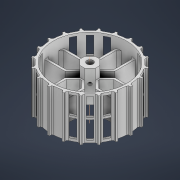
# Autodesk Inventor part: Reifen_v2
Saved by Autodesk Inventor 2021 (Build 250183000, 183)
## iProperties
Created: 2021-01-03
Part Number: Reifen_v2
Material: Generisch
Document SubType Name: Modeling
Designer: Ctroi
Density: 1 g/cm^3
Appearance: Vorgabe
Author: Ctroi
## iProperties of the stored document _3D-Druck.ipt
Created: 2021-01-03
Part Number: _3D-Druck
Material: Generisch
Document SubType Name: Modeling
Designer: Ctroi
Density: 1 g/cm^3
Appearance: Vorgabe
Author: Ctroi
Autodesk Inventor part; units mm, degrees
ref_plane "YZ Plane" through (0, 0, 0) normal (1, 0, 0) x (0, 1, 0)
ref_plane "XZ Plane" through (0, 0, 0) normal (0, 1, 0) x (-1, 0, 0)
ref_plane "XY Plane" through (0, 0, 0) normal (0, 0, 1) x (1, 0, 0)
sketch "Grundskizze" plane through (0, 0, 0) normal (0, 1, 0) x (-1, 0, 0)
  circle A0 centre (0, 0) radius 55
  circle A1 centre (0, 0) radius 52
  circle A2 centre (0, 0) radius 4.5
  line L0 (11, -3.1421) -> (3.1421, -11)
  line L1 (-3.1421, -11) -> (-11, -3.1421)
  line L2 (-11, 3.1421) -> (-3.1421, 11)
  line L3 (3.1421, 11) -> (11, 3.1421)
  line L4 (0, -77) -> (0, 77) projected
  line L5 (77, 0) -> (-77, 0) projected
  line L6 (3.1421, -11) -> (-3.1421, -11)
  line L7 (-11, -3.1421) -> (-11, 3.1421)
  line L8 (-3.1421, 11) -> (3.1421, 11)
  line L9 (11, 3.1421) -> (11, -3.1421)
  line L10 (3.1421, -11) -> (13.7487, -21.6066)
  line L11 (3.1421, -11) -> (18.1421, -11) construction
  line L12 (13.7487, -21.6066) -> (13.7487, -50.1495)
  line L13 (-3.1421, -11) -> (-13.7487, -21.6066)
  line L14 (-3.1421, -11) -> (11.8579, -11) construction
  line L15 (-13.7487, -21.6066) -> (-13.7487, -50.1495)
  line L16 (10.7487, -44.9441) -> (10.7487, -22.8492)
  line L17 (10.7487, -22.8492) -> (1.0208, -13.1213)
  line L18 (-10.7487, -44.4688) -> (-10.7487, -22.8492)
  line L19 (-10.7487, -22.8492) -> (-1.0208, -13.1213)
  line L20 (1.0208, -13.1213) -> (-1.0208, -13.1213)
  line L21 (10.7487, -44.9441) -> (10.7487, -50.877)
  line L22 (-10.7487, -44.4688) -> (-10.7487, -50.877)
  line L23 (21.6066, -13.7487) -> (50.1495, -13.7487)
  line L24 (44.4688, -10.7487) -> (50.877, -10.7487)
  line L25 (44.4688, -10.7487) -> (22.8492, -10.7487)
  line L26 (22.8492, -10.7487) -> (13.1213, -1.0208)
  line L27 (11, -3.1421) -> (21.6066, -13.7487)
  line L28 (22.8492, 10.7487) -> (13.1213, 1.0208)
  line L29 (13.1213, 1.0208) -> (13.1213, -1.0208)
  line L30 (11, 3.1421) -> (21.6066, 13.7487)
  line L31 (44.9441, 10.7487) -> (22.8492, 10.7487)
  line L32 (21.6066, 13.7487) -> (50.1495, 13.7487)
  line L33 (44.9441, 10.7487) -> (50.877, 10.7487)
  line L34 (13.7487, 21.6066) -> (13.7487, 50.1495)
  line L35 (10.7487, 44.4688) -> (10.7487, 50.877)
  line L36 (10.7487, 44.4688) -> (10.7487, 22.8492)
  line L37 (10.7487, 22.8492) -> (1.0208, 13.1213)
  line L38 (3.1421, 11) -> (13.7487, 21.6066)
  line L39 (-10.7487, 22.8492) -> (-1.0208, 13.1213)
  line L40 (-1.0208, 13.1213) -> (1.0208, 13.1213)
  line L41 (-3.1421, 11) -> (-13.7487, 21.6066)
  line L42 (-10.7487, 44.9441) -> (-10.7487, 22.8492)
  line L43 (-13.7487, 21.6066) -> (-13.7487, 50.1495)
  line L44 (-10.7487, 44.9441) -> (-10.7487, 50.877)
  line L45 (-21.6066, 13.7487) -> (-50.1495, 13.7487)
  line L46 (-44.4688, 10.7487) -> (-50.877, 10.7487)
  line L47 (-44.4688, 10.7487) -> (-22.8492, 10.7487)
  line L48 (-22.8492, 10.7487) -> (-13.1213, 1.0208)
  line L49 (-11, 3.1421) -> (-21.6066, 13.7487)
  line L50 (-22.8492, -10.7487) -> (-13.1213, -1.0208)
  line L51 (-13.1213, -1.0208) -> (-13.1213, 1.0208)
  line L52 (-11, -3.1421) -> (-21.6066, -13.7487)
  line L53 (-44.9441, -10.7487) -> (-22.8492, -10.7487)
  line L54 (-21.6066, -13.7487) -> (-50.1495, -13.7487)
  line L55 (-44.9441, -10.7487) -> (-50.877, -10.7487)
  line L56 (-10.7487, -47.6729) -> (-7.4827, -51.4588)
  line L57 (-7.4827, -51.4588) -> (-10.7487, -51.4588)
  line L58 (-10.7487, -51.4588) -> (-10.7487, -47.6729)
  line L59 (10.7487, -47.6729) -> (7.4827, -51.4588)
  line L60 (7.4827, -51.4588) -> (10.7487, -51.4588)
  line L61 (10.7487, -51.4588) -> (10.7487, -47.6729)
  line L62 (51.4588, -10.7487) -> (47.6729, -10.7487)
  line L63 (47.6729, -10.7487) -> (51.4588, -7.4827)
  line L64 (51.4588, -7.4827) -> (51.4588, -10.7487)
  line L65 (51.4588, 10.7487) -> (47.6729, 10.7487)
  line L66 (47.6729, 10.7487) -> (51.4588, 7.4827)
  line L67 (51.4588, 7.4827) -> (51.4588, 10.7487)
  circle A3 centre (0, 0) radius 4.5
  line L68 (10.7487, 51.4588) -> (10.7487, 47.6729)
  line L69 (10.7487, 47.6729) -> (7.4827, 51.4588)
  line L70 (7.4827, 51.4588) -> (10.7487, 51.4588)
  line L71 (-10.7487, 51.4588) -> (-10.7487, 47.6729)
  line L72 (-10.7487, 47.6729) -> (-7.4827, 51.4588)
  line L73 (-7.4827, 51.4588) -> (-10.7487, 51.4588)
  circle A4 centre (0, 0) radius 4.5
  line L74 (-51.4588, 10.7487) -> (-47.6729, 10.7487)
  line L75 (-47.6729, 10.7487) -> (-51.4588, 7.4827)
  line L76 (-51.4588, 7.4827) -> (-51.4588, 10.7487)
  line L77 (-51.4588, -10.7487) -> (-47.6729, -10.7487)
  line L78 (-47.6729, -10.7487) -> (-51.4588, -7.4827)
  line L79 (-51.4588, -7.4827) -> (-51.4588, -10.7487)
  circle A5 centre (0, 0) radius 4.5
  point P0 (0, -11)
  point P1 (-50.1495, 13.7487)
  point P2 (-50.877, 10.7487)
  point P3 (-50.1495, -13.7487)
  point P4 (13.7487, 50.1495)
  point P5 (10.7487, 50.877)
  point P6 (-13.7487, 50.1495)
  point P7 (50.877, -10.7487)
  point P8 (50.877, 10.7487)
  point P9 (50.1495, 13.7487)
  point P10 (50.877, 10.7487)
  point P11 (10.7487, 50.877)
  point P12 (-10.7487, 50.877)
  point P13 (-50.877, 10.7487)
  point P14 (-50.877, -10.7487)
  dimension "d0" = 110
  dimension "d1" = 3
  dimension "d2" = 9
  dimension "d7" = 15
  dimension "d8" = 45
  dimension "d10" = 135
  dimension "d11" = 3
  dimension "d12" = 3
  dimension "d52" = 360
  dimension "d88" = 5
  dimension "d91" = 360
  dimension "d93" = 40.784
  constraints: 156 end point, 6 centre point, 6 vertical, 5 horizontal, 5 point on circle, 4 coincident, 4 parallel, 4 perpendicular, 3 symmetric about line, 2 equal length, 2 midpoint, 1 point on line, 174 other
  measures "d0" diameter of A0
  measures "d1" radial gap between concentric circles of A0 A1
  measures "d2" diameter of A2
  measures "d7" distance of L0.end L10.end
  measures "d8" angle of L10 L11
  measures "d10" angle of L13 L14
  measures "d11" distance between parallel lines of L12 L16
  measures "d12" distance between parallel lines of L15 L18
  measures "d88" distance of L56.start L56.end
  measures "d93" angle of L56 L22
extrude "Außenrahmen" add sketch "Grundskizze" along normal blind 45 and the other way blind 15 contours L5 A1 L67 L65 L68 L70 L4 A0 | A0 L4 A1 L60 L61 L62 L64 L5 | L4 A1 L73 L71 L74 L76 L5 A0 | A0 L5 A1 L79 L77 L58 L57 L4 | A1 L65 L67 | L64 L62 A1 | L70 L68 A1 | A1 L71 L73 | L57 L58 A1 | A1 L61 L60 | L76 L74 A1 | A1 L77 L79
extrude "Radnabe" add sketch "Grundskizze" along normal blind 45 contours L9 L0 L6 L4 A2 L5 | L5 A2 L4 L8 L3 L9 | L4 A2 L5 L7 L2 L8 | L6 L1 L7 L5 A2 L4
sketch "Profilskizze" plane through (0, 45, 0) normal (0, 1, 0) x (1, 0, 0)
  circle A0 centre (0, 0) radius 55 projected
  circle A1 centre (0, 0) radius 55 projected
  line L0 (1.5, 54.9795) -> (1.5, 58.5)
  line L1 (1, 59) -> (-1, 59)
  line L2 (-1.5, 58.5) -> (-1.5, 54.9795)
  line L3 (0, 81.9243) -> (0, -77.8207) projected
  arc A2 (-1, 59) -> (-1.5, 58.5) centre (-1, 58.5) ccw
  arc A3 (1.5, 58.5) -> (1, 59) centre (1, 58.5) ccw
  line L4 (-1.5, 54.9795) -> (-1.5, 56.4795)
  line L5 (-1.5, 56.4795) -> (-3.4319, 54.8928)
  line L6 (-3.4319, 54.8928) -> (-1.5, 54.9795)
  line L7 (1.5, 54.9795) -> (1.5, 56.4795)
  line L8 (1.5, 56.4795) -> (3.4319, 54.8928)
  line L9 (3.4319, 54.8928) -> (1.5, 54.9795)
  point P0 (1.5, 59)
  point P1 (-1.5, 59)
  dimension "d58" = 0.5
  dimension "d64" = 4
  dimension "d65" = 3
  dimension "d78" = 1.5
  dimension "d79" = 2.5
  constraints: 18 end point, 7 point on circle, 5 point on line, 4 tangent, 2 centre point, 2 horizontal alignment, 2 parallel, 1 equal radius, 1 other
  measures "d58" radius of A2
  measures "d64" distance edge to line of A0 L1
  measures "d65" distance between parallel lines of L2 L0
  measures "d78" distance of L2.end L4.end
  measures "d79" distance of L4.end L5.end
extrude "Streben" add sketch "Grundskizze" along normal blind 30 contours L66 L33 A1 | L64 L62 A1 | A1 L24 L63 | L29 L26 L25 L24 A1 L23 L27 L9 L5 | L5 L9 L30 L32 A1 L33 L31 L28 L29 | A1 L35 L69 | L72 L44 A1 | A1 L71 L73 | L40 L37 L36 L35 A1 L34 L38 L8 L4 | L4 L8 L41 L43 A1 L44 L42 L39 L40 | A1 L22 L56 | L59 L21 A1 | A1 L61 L60 | L20 L19 L18 L22 A1 L15 L13 L6 L4 | L4 L6 L10 L12 A1 L21 L16 L17 L20 | L76 L74 A1 | A1 L46 L75 | L78 L55 A1 | L51 L48 L47 L46 A1 L45 L49 L7 L5 | L5 L7 L52 L54 A1 L55 L53 L50 L51
extrude "Profil" add sketch "Profilskizze" against normal blind 60 contours A0 L0 L8 | A0 L3 L1 A3 L0 | L5 L2 A0 | A0 L2 A2 L1 L3
pattern_circular "Runde Anordnung1" count 20 over 360 about axis through (0, 0, 0) along (0, 1, 0) of "Profil"
sketch "Einpresssmutter_skizze" plane through (-11, 0, -3.1421) normal (-0.7071068, 0, -0.7071068) x (-0.7071068, 0, 0.7071068)
  circle A0 centre (-5.5563, 25.6612) radius 2.25
  line L0 (-12.6755, -15) -> (-12.6755, 45) projected
  line L1 (-0.0311, 45) -> (-0.0311, 0)
  line L2 (-11.1127, 45) -> (-15.5563, 45) projected
  line L3 (-11.1127, 45) -> (-11.1127, 0)
  point P0 (-5.5563, 0)
  dimension "d71" = 4.5
  dimension "d72" = 7.1192
  constraints: 4 end point, 2 vertical, 1 centre point
  measures "d71" diameter of A0
  measures "d72" distance from line of L0 A0.centre
extrude "Loch Einpressmutter 1" cut sketch "Einpresssmutter_skizze" against normal up to surface round surface about axis through (0, 0, 0) along (0, 1, 0) radius 4.5 far side no
sketch "Einpressmutter_skizze2" plane through (11, 0, 3.1421) normal (0.7071068, 0, 0.7071068) x (0.7071068, 0, -0.7071068)
  circle A0 centre (-5.5563, 25.6726) radius 2.25
  point P0 (-5.5563, 0)
  dimension "d75" = 4.5
  constraints: 1 centre point
  measures "d75" diameter of A0
extrude "Loch Einpressmutter 2" cut sketch "Einpressmutter_skizze2" against normal up to surface round surface about axis through (0, 0, 0) along (0, 1, 0) radius 4.5 far side no
ref_plane "Arbeitsebene2" through (38.8909, -15, -38.8909) normal (0.7071068, 0, -0.7071068) x (0, 1, 0)
sketch "Skizze9" plane through (38.8909, -15, -38.8909) normal (0.7071068, 0, -0.7071068) x (0, 1, 0)
  line L0 (3.5, 3.75) -> (28.5, 3.75)
  line L1 (28.5, 3.75) -> (28.5, -3.75)
  line L2 (28.5, -3.75) -> (3.5, -3.75)
  line L3 (3.5, -3.75) -> (3.5, 3.75)
  line L4 (31.5, 3.75) -> (56.5, 3.75)
  line L5 (56.5, 3.75) -> (56.5, -3.75)
  line L6 (56.5, -3.75) -> (31.5, -3.75)
  line L7 (31.5, -3.75) -> (31.5, 3.75)
  line L8 (-12, 0) -> (72, 0) projected
  line L9 (0, 5.1975) -> (0, -5.1975) projected
  line L10 (60, -5.1975) -> (60, 5.1975) projected
  line L11 (3.5, -13.25) -> (28.5, -13.25)
  line L12 (3.5, -20.75) -> (3.5, -13.25)
  line L13 (28.5, -20.75) -> (3.5, -20.75)
  line L14 (28.5, -13.25) -> (28.5, -20.75)
  line L15 (31.5, -13.25) -> (56.5, -13.25)
  line L16 (31.5, -20.75) -> (31.5, -13.25)
  line L17 (56.5, -20.75) -> (31.5, -20.75)
  line L18 (56.5, -13.25) -> (56.5, -20.75)
  line L19 (3.5, 20.75) -> (28.5, 20.75)
  line L20 (3.5, 13.25) -> (3.5, 20.75)
  line L21 (28.5, 13.25) -> (3.5, 13.25)
  line L22 (28.5, 20.75) -> (28.5, 13.25)
  line L23 (31.5, 20.75) -> (56.5, 20.75)
  line L24 (31.5, 13.25) -> (31.5, 20.75)
  line L25 (56.5, 13.25) -> (31.5, 13.25)
  line L26 (56.5, 20.75) -> (56.5, 13.25)
  point P0 (15, 0)
  dimension "d107" = 25
  dimension "d108" = 7.5
  dimension "d109" = 25
  dimension "d110" = 7.5
  dimension "d111" = 3.5
  dimension "d112" = 3.5
  dimension "d115" = 17
  dimension "d122" = 17
  constraints: 48 end point, 4 parallel, 2 horizontal, 2 perpendicular, 2 vertical, 34 other
  measures "d107" distance of L1.end L2.end
  measures "d108" distance of L0.end L1.end
  measures "d109" distance of L5.end L6.end
  measures "d110" distance of L4.end L5.end
  measures "d111" distance between parallel lines of L3 L9
  measures "d112" distance between parallel lines of L5 L10
  measures "d115" distance of L0.start L11.start
  measures "d122" distance of L0.start L19.start
extrude "Extrusion13" cut sketch "Skizze9" against normal mid plane 16
pattern_circular "Runde Anordnung4" count 4 over 360 about axis through (0, 0, 0) along (0, 1, 0) of "Extrusion13"
